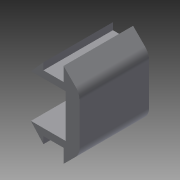
# Autodesk Inventor part: clema cablu profil
Saved by Autodesk Inventor 2015 SP1 (Build 190203100, 203)
## iProperties
Created: 2015-08-08
Part Number: clema cablu profil
Material: Generic
Document SubType Name: Modeling
Designer: ubik
Density: 1 g/cm^3
Appearance: Default
Author: ubik
Autodesk Inventor part; units mm, degrees
ref_plane "YZ Plane" through (0, 0, 0) normal (1, 0, 0) x (0, 1, 0)
ref_plane "XZ Plane" through (0, 0, 0) normal (0, 1, 0) x (-1, 0, 0)
ref_plane "XY Plane" through (0, 0, 0) normal (0, 0, 1) x (1, 0, 0)
sketch "Sketch1" plane through (0, 0, 0) normal (0, 0, 1) x (1, 0, 0)
  line L0 (15, -4.1) -> (12.1, -4.1)
  line L1 (12.1, 4.1) -> (15, 4.1)
  line L2 (12.1, 4.1) -> (12.1, 5.1)
  line L3 (10.3015, 3.1) -> (12.1, 5.1)
  line L4 (10.3015, -3.1) -> (12.1, -5.1)
  line L5 (12.1, -5.1) -> (12.1, -4.1)
  line L6 (15.3015, 3.1) -> (15.3015, -3.1)
  line L7 (15, 4.1) -> (15, 6.1)
  line L8 (15, 6.1) -> (16.7157, 4.3843)
  line L9 (15, -4.1) -> (15, -6.1)
  line L10 (15, -6.1) -> (16.7157, -4.3843)
  line L11 (17.3015, 2.97) -> (17.3015, -2.97)
  line L12 (15.3015, 3.1) -> (10.3015, 3.1)
  line L13 (15.3015, -3.1) -> (10.3015, -3.1)
  arc A0 (17.3015, 2.97) -> (16.7157, 4.3843) centre (15.3015, 2.97) ccw
  arc A1 (16.7157, -4.3843) -> (17.3015, -2.97) centre (15.3015, -2.97) ccw
  point P0 (0, 0)
  point P1 (17.3015, 3.7985)
  point P2 (17.3015, -3.7985)
  dimension "d0" = 1
  dimension "d2" = 45
  dimension "d3" = 45
  dimension "d4" = 2.3015
  dimension "d5" = 2.3015
  dimension "d6" = 2
  dimension "d7" = 2
  dimension "d8" = 1
  dimension "d9" = 1
  dimension "d10" = 5
  dimension "d11" = 5
  dimension "d12" = 1
  dimension "d13" = 2
  dimension "d16" = 2.9
  dimension "d17" = 2.9
  dimension "d18" = 2
  constraints: 28 end point, 4 point on circle, 4 point on line, 4 tangent, 3 vertical, 2 centre point, 2 horizontal, 2 perpendicular, 1 equal radius
  measures "d0" distance of L1.start L2.end
  measures "d2" angle of L7 L8
  measures "d3" angle of L10 L9
  measures "d4" horizontal distance of L7.end point (17.301, 3.798)
  measures "d5" horizontal distance of L9.end point (17.301, -3.798)
  measures "d6" distance of L1.end L7.end
  measures "d7" distance of L0.start L9.end
  measures "d8" distance between parallel lines of L1 L12
  measures "d9" distance between parallel lines of L0 L13
  measures "d10" distance of L6.start L3.start
  measures "d11" distance of L6.end L4.start
  measures "d12" distance of L4.end L0.end
  measures "d13" radius of A0
  measures "d16" distance of L1.start L1.end
  measures "d17" distance of L0.start L0.end
  measures "d18" distance between parallel lines of L11 L6
extrude "Extrusion1" add sketch "Sketch1" along normal blind 10
equation "\"d5\" = d4"
equation "\"d7\" = d6"
equation "\"d9\" = d8"
equation "\"d11\" = d10"
equation "\"d12\" = d0"
equation "\"d17\" = d16"
body "Solid1"
